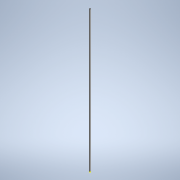
# Autodesk Inventor part: wood spar
Saved by Autodesk Inventor 2021 (Build 250183000, 183)
## iProperties
Created: 2021-03-06
Part Number: wood spar
Material: Generic
Document SubType Name: Modeling
Designer: Ferdinand Hubbard
Density: 1 g/cm^3
Appearance: Default
Author: Ferdinand Hubbard
Autodesk Inventor part; units mm, degrees
ref_plane "YZ Plane" through (0, 0, 0) normal (1, 0, 0) x (0, 1, 0)
ref_plane "XZ Plane" through (0, 0, 0) normal (0, 1, 0) x (-1, 0, 0)
ref_plane "XY Plane" through (0, 0, 0) normal (0, 0, 1) x (1, 0, 0)
sketch "Sketch1" plane through (0, 0, 0) normal (0, 1, 0) x (-1, 0, 0)
  line L0 (0, 0) -> (-13, 0)
  line L1 (-13, 0) -> (-13, -13)
  line L2 (-13, -13) -> (0, -13)
  line L3 (0, -13) -> (0, 0)
  dimension "d0" = 13
  dimension "d1" = 13
  constraints: 8 end point, 2 parallel, 1 horizontal, 1 perpendicular
  measures "d0" distance of L2.end L1.end
  measures "d1" distance of L1.end L0.end
extrude "Extrusion1" add sketch "Sketch1" along normal blind 2000
sketch "Sketch2" plane through (13, 0, -13) normal (1, 0, 0) x (0, 0, -1)
  point P0 (-13, 0)
body "Solid1"
